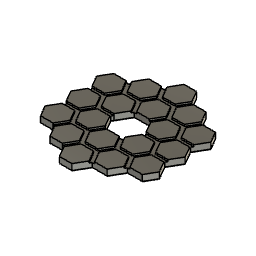
Mirror-v03 v3 (Autodesk Fusion 360 design; units mm, degrees)
Autodesk Fusion 360 part; units mm, degrees
sketch "Skizze1" plane through (0, 0, 0) normal (0, 0, 1) x (1, 0, 0)
  line L0 (8.3699, -6.8911) -> (9.0627, -6.8911)
  line L1 (23.8717, -11.2411) -> (21.7067, -7.4911) construction
  line L2 (4.3862, -7.4911) -> (2.2211, -11.2411) construction
  line L3 (21.0139, -7.4911) -> (21.3603, -8.0911)
  line L4 (21.3603, -6.8911) -> (23.1789, -3.7411)
  line L5 (17.723, -6.8911) -> (21.3603, -6.8911) construction
  line L6 (10.8814, -3.7411) -> (8.7163, -7.4911) construction
  line L7 (11.2278, -3.1411) -> (14.8651, -3.1411) construction
  line L8 (15.2115, -3.7411) -> (10.8814, -3.7411) construction
  line L9 (16.6837, -7.4911) -> (14.8651, -4.3411) construction
  line L10 (21.3603, -8.0911) -> (17.723, -8.0911) construction
  line L11 (17.3765, -7.4911) -> (21.7067, -7.4911) construction
  line L12 (21.7067, -7.4911) -> (23.8717, -3.7411) construction
  line L13 (10.8814, -3.7411) -> (15.2115, -3.7411) construction
  line L14 (-3.5813, -7.4911) -> (-1.7626, -10.6411) construction
  line L15 (9.4091, -7.4911) -> (9.0627, -6.8911)
  line L16 (17.3765, -7.4911) -> (15.2115, -3.7411) construction
  line L17 (21.3603, -6.8911) -> (21.0139, -7.4911)
  line L18 (8.7163, -7.4911) -> (10.8814, -11.2411) construction
  line L19 (14.8651, -4.3411) -> (11.2278, -4.3411) construction
  line L20 (21.7067, -7.4911) -> (17.3765, -7.4911) construction
  line L21 (9.4091, -7.4911) -> (11.2278, -10.6411)
  line L22 (15.2115, -3.7411) -> (17.3765, -7.4911) construction
  line L23 (8.7163, -7.4911) -> (10.8814, -3.7411) construction
  line L24 (1.8747, -10.6411) -> (3.6933, -7.4911)
  line L25 (15.9043, -3.7411) -> (17.723, -6.8911) construction
  line L26 (-2.109, -11.2411) -> (-4.2741, -7.4911) construction
  line L27 (14.8651, -10.6411) -> (16.6837, -7.4911) construction
  line L28 (10.8814, 3.7589) -> (8.7163, 0.0089) construction
  line L29 (-8.2578, -8.0911) -> (-10.0765, -11.2411)
  line L30 (17.723, -8.0911) -> (15.9043, -11.2411) construction
  line L31 (2.2211, -11.2411) -> (4.3862, -7.4911) construction
  line L32 (17.3765, -7.4911) -> (15.2115, -11.2411) construction
  line L33 (8.7163, 7.5089) -> (4.3862, 7.5089) construction
  line L34 (-8.6042, -7.4911) -> (-10.7693, -11.2411) construction
  line L35 (10.1885, 3.7589) -> (8.3699, 6.9089)
  line L36 (10.8814, -11.2411) -> (8.7163, -7.4911) construction
  line L37 (8.7163, -7.4911) -> (4.3862, -7.4911) construction
  line L38 (8.3699, -15.5911) -> (4.7326, -15.5911)
  line L39 (17.723, -0.5911) -> (15.9043, -3.7411) construction
  line L40 (8.7163, -22.4911) -> (4.3862, -22.4911) construction
  line L41 (4.3862, 0.0089) -> (8.7163, 0.0089) construction
  line L42 (4.7326, -21.8911) -> (8.3699, -21.8911) construction
  line L43 (4.7326, -6.8911) -> (8.3699, -6.8911)
  line L44 (9.4091, 0.0089) -> (11.2278, -3.1411) construction
  line L45 (10.8814, -3.7411) -> (8.7163, 0.0089) construction
  line L46 (4.3862, -22.4911) -> (8.7163, -22.4911) construction
  line L47 (8.3699, -23.0911) -> (4.7326, -23.0911) construction
  line L48 (23.1789, -3.7411) -> (21.3603, -0.5911)
  line L49 (10.1885, -3.7411) -> (8.3699, -0.5911) construction
  line L50 (11.2278, -10.6411) -> (11.5742, -11.2411)
  line L51 (-2.109, -18.7411) -> (-4.2741, -14.9911) construction
  line L52 (-2.8018, -18.7411) -> (-4.6205, -15.5911) construction
  line L53 (21.0139, -14.9911) -> (21.3603, -15.5911)
  line L54 (3.6933, -7.4911) -> (1.8747, -4.3411) construction
  line L55 (23.1789, -18.7411) -> (21.3603, -15.5911)
  line L56 (-4.2741, -14.9911) -> (-8.6042, -14.9911) construction
  line L57 (21.3603, -15.5911) -> (17.723, -15.5911) construction
  line L58 (17.3765, -14.9911) -> (15.2115, -11.2411) construction
  line L59 (15.9043, -11.2411) -> (17.723, -14.3911) construction
  line L60 (4.3759, -14.9895) -> (2.2081, -11.2411) construction
  line L61 (4.7326, -6.8911) -> (4.0398, -6.8911)
  line L62 (1.8595, -11.8154) -> (-1.7778, -11.8154) construction
  line L63 (17.3765, -22.4911) -> (21.7067, -22.4911) construction
  line L64 (-8.2578, -15.5911) -> (-10.0765, -18.7411)
  line L65 (4.3677, -22.5014) -> (2.2026, -18.7514) construction
  line L66 (16.6837, -14.9911) -> (14.8651, -11.8411) construction
  line L67 (8.7163, -14.9911) -> (10.8814, -18.7411) construction
  line L68 (8.3699, -29.3911) -> (10.1885, -26.2411)
  line L69 (4.3862, -7.4911) -> (2.2211, -3.7411) construction
  line L70 (10.1885, -26.2411) -> (8.3699, -23.0911) construction
  line L71 (8.7163, -14.9911) -> (10.8814, -11.2411) construction
  line L72 (14.8651, -25.6411) -> (16.6837, -22.4911)
  line L73 (17.723, -14.3911) -> (21.3603, -14.3911) construction
  line L74 (10.8814, -18.7411) -> (8.7163, -14.9911) construction
  line L75 (2.9139, -3.7411) -> (4.7326, -6.8911) construction
  line L76 (14.8651, -18.1411) -> (16.6837, -14.9911) construction
  line L77 (15.2115, -26.2411) -> (17.3765, -22.4911) construction
  line L78 (17.723, -15.5911) -> (15.9043, -18.7411) construction
  line L79 (-8.2578, -15.5911) -> (-7.9114, -14.9911)
  line L80 (1.8154, -18.1524) -> (3.6663, -14.948) construction
  line L81 (17.723, -21.8911) -> (21.3603, -21.8911)
  line L82 (21.3603, -14.3911) -> (23.1789, -11.2411)
  line L83 (10.1885, -26.2411) -> (10.5349, -25.6411)
  line L84 (9.4091, -22.4911) -> (11.2278, -25.6411) construction
  line L85 (17.0301, -21.8911) -> (16.6837, -22.4911)
  line L86 (-8.6042, 0.0089) -> (-10.7693, -3.7411) construction
  line L87 (4.7326, -15.5911) -> (4.0398, -15.5911)
  line L88 (8.7163, -29.9911) -> (10.8814, -26.2411) construction
  line L89 (11.2278, -25.6411) -> (10.5349, -25.6411)
  line L90 (-4.2741, 0.0089) -> (-2.109, -3.7411) construction
  line L91 (17.3765, -22.4911) -> (15.2115, -18.7411) construction
  line L92 (11.2278, -11.8411) -> (11.5742, -11.2411)
  line L93 (8.7163, -22.4911) -> (10.8814, -26.2411) construction
  line L94 (8.3699, -15.5911) -> (9.0627, -15.5911)
  line L95 (1.8747, -10.6411) -> (1.5282, -11.2411)
  line L96 (17.3765, -14.9911) -> (15.2115, -18.7411) construction
  line L97 (3.6933, -7.4911) -> (4.0398, -6.8911)
  line L98 (4.3862, 0.0089) -> (2.2211, -3.7411) construction
  line L99 (3.6663, -14.948) -> (1.8595, -11.8154)
  line L100 (2.2127, -18.7479) -> (4.3759, -14.9895) construction
  line L101 (10.8814, -26.2411) -> (8.7163, -22.4911) construction
  line L102 (2.2211, -3.7411) -> (4.3862, -7.4911) construction
  line L103 (15.2115, -18.7411) -> (17.3765, -22.4911) construction
  line L104 (15.2115, -11.2411) -> (17.3765, -14.9911) construction
  line L105 (-8.2578, -0.5911) -> (-10.0765, -3.7411)
  line L106 (17.3765, -14.9911) -> (21.7067, -14.9911) construction
  line L107 (-2.109, -11.2411) -> (2.2211, -11.2411) construction
  line L108 (2.2081, -11.2411) -> (-2.096, -11.2411) construction
  line L109 (11.2278, -18.1411) -> (14.8651, -18.1411) construction
  line L110 (-8.6042, -14.9911) -> (-10.7693, -18.7411) construction
  line L111 (11.2278, -19.3411) -> (9.4091, -22.4911) construction
  line L112 (2.2211, -11.2411) -> (4.3862, -14.9911) construction
  line L113 (9.4091, -14.9911) -> (11.2278, -18.1411) construction
  line L114 (14.8651, -3.1411) -> (16.6837, 0.0089) construction
  line L115 (4.7326, 0.6089) -> (8.3699, 0.6089) construction
  line L116 (-3.6204, -15.0117) -> (-1.8049, -18.1518) construction
  line L117 (14.8651, -19.3411) -> (11.2278, -19.3411) construction
  line L118 (23.8717, -3.7411) -> (21.7067, 0.0089) construction
  line L119 (8.3699, -0.5911) -> (4.7326, -0.5911) construction
  line L120 (4.7326, -29.3911) -> (8.3699, -29.3911)
  line L121 (4.7326, -15.5911) -> (2.9139, -18.7411) construction
  line L122 (10.8814, -11.2411) -> (8.7163, -14.9911) construction
  line L123 (10.1885, -18.7411) -> (8.3699, -15.5911) construction
  line L124 (4.3862, -29.9911) -> (8.7163, -29.9911) construction
  line L125 (8.3699, 6.9089) -> (4.7326, 6.9089)
  line L126 (8.7163, 0.0089) -> (10.8814, -3.7411) construction
  line L127 (14.8651, -11.8411) -> (11.2278, -11.8411) construction
  line L128 (10.8814, -18.7411) -> (8.7163, -22.4911) construction
  line L129 (11.2278, -11.8411) -> (9.4091, -14.9911)
  line L130 (-2.8018, -3.7411) -> (-4.6205, -0.5911) construction
  line L131 (1.8747, -3.1411) -> (3.6933, 0.0089) construction
  line L132 (23.8717, -18.7411) -> (21.7067, -14.9911) construction
  line L133 (15.2115, -18.7411) -> (10.8814, -18.7411) construction
  line L134 (10.8814, -18.7411) -> (15.2115, -18.7411) construction
  line L135 (-4.2836, -15.045) -> (-2.1376, -18.7549) construction
  line L136 (11.2278, -10.6411) -> (14.8651, -10.6411) construction
  line L137 (15.2115, -3.7411) -> (17.3765, 0.0089) construction
  line L138 (11.2278, -25.6411) -> (14.8651, -25.6411)
  line L139 (8.3699, -21.8911) -> (10.1885, -18.7411) construction
  line L140 (1.8595, -11.8154) -> (1.5282, -11.2411)
  line L141 (8.7163, -22.4911) -> (10.8814, -18.7411) construction
  line L142 (9.0627, -15.5911) -> (9.4091, -14.9911)
  line L143 (3.6663, -14.948) -> (4.0398, -15.5911)
  line L144 (8.7163, -14.9911) -> (4.3862, -14.9911) construction
  line L145 (4.3862, -14.9911) -> (2.2211, -18.7411) construction
  line L146 (10.8814, -26.2411) -> (15.2115, -26.2411) construction
  line L147 (10.8814, -11.2411) -> (15.2115, -11.2411) construction
  line L148 (8.7163, 0.0089) -> (4.3862, 0.0089) construction
  line L149 (2.2211, -3.7411) -> (4.3862, 0.0089) construction
  line L150 (4.3862, -7.4911) -> (8.7163, -7.4911) construction
  line L151 (4.3862, -14.9911) -> (8.7163, -14.9911) construction
  line L152 (15.2115, -11.2411) -> (10.8814, -11.2411) construction
  line L153 (17.3765, 0.0089) -> (15.2115, -3.7411) construction
  line L154 (-2.109, -3.7411) -> (-4.2741, -7.4911) construction
  line L155 (-10.7693, -11.2411) -> (-8.6042, -14.9911) construction
  line L156 (4.7326, -0.5911) -> (2.9139, -3.7411) construction
  line L157 (-8.2578, -6.8911) -> (-7.9114, -7.4911)
  line L158 (4.3862, 0.0089) -> (2.2211, 3.7589) construction
  line L159 (-2.1275, -26.2514) -> (2.2026, -26.2514) construction
  line L160 (-1.8049, -18.1518) -> (1.8154, -18.1524) construction
  line L161 (21.3603, -21.8911) -> (23.1789, -18.7411)
  line L162 (4.3862, -22.4911) -> (2.2211, -26.2411) construction
  line L163 (-8.6042, -14.9911) -> (-4.2741, -14.9911) construction
  line L164 (-4.6205, -15.5911) -> (-8.2578, -15.5911) construction
  line L165 (-1.7778, -11.8154) -> (-3.6204, -15.0117) construction
  line L166 (-10.0765, -11.2411) -> (-8.2578, -14.3911)
  line L167 (15.2115, -18.7411) -> (17.3765, -14.9911) construction
  line L168 (-4.2741, -22.4911) -> (-2.109, -18.7411) construction
  line L169 (-2.096, -11.2411) -> (-4.2836, -15.045) construction
  line L170 (15.9043, -18.7411) -> (17.723, -21.8911) construction
  line L171 (-10.0765, -3.7411) -> (-8.2578, -6.8911)
  line L172 (21.7067, -14.9911) -> (17.3765, -14.9911) construction
  line L173 (1.8747, -4.3411) -> (-1.7626, -4.3411) construction
  line L174 (2.2211, -3.7411) -> (-2.109, -3.7411) construction
  line L175 (-4.2741, -7.4911) -> (-8.6042, -7.4911) construction
  line L176 (17.723, -21.8911) -> (17.0301, -21.8911)
  line L177 (2.2211, -26.2411) -> (4.3862, -29.9911) construction
  line L178 (-4.6205, -8.0911) -> (-8.2578, -8.0911) construction
  line L179 (-1.7726, -25.6367) -> (1.8478, -25.6367)
  line L180 (21.7067, -22.4911) -> (23.8717, -18.7411) construction
  line L181 (-7.9114, -14.9911) -> (-8.2578, -14.3911)
  line L182 (-1.7626, -10.6411) -> (1.8747, -10.6411) construction
  line L183 (-3.5813, 0.0089) -> (-1.7626, -3.1411) construction
  line L184 (-3.5828, -22.5014) -> (-1.7726, -25.6367)
  line L185 (-4.2741, -14.9911) -> (-2.109, -11.2411) construction
  line L186 (-2.1376, -18.7549) -> (2.2127, -18.7479) construction
  line L187 (21.7067, -14.9911) -> (23.8717, -11.2411) construction
  line L188 (2.9139, -26.2411) -> (4.7326, -29.3911)
  line L189 (-2.109, -3.7411) -> (2.2211, -3.7411) construction
  line L190 (3.6579, -22.5014) -> (1.8478, -19.366) construction
  line L191 (1.8478, -25.6367) -> (3.6579, -22.5014) construction
  line L192 (-8.2578, -21.8911) -> (-4.6205, -21.8911)
  line L193 (-4.6205, -21.8911) -> (-2.8018, -18.7411) construction
  line L194 (2.2211, -18.7411) -> (4.3862, -22.4911) construction
  line L195 (16.6837, -22.4911) -> (14.8651, -19.3411) construction
  line L196 (-1.7626, -4.3411) -> (-3.5813, -7.4911) construction
  line L197 (1.8478, -19.366) -> (-1.7726, -19.366) construction
  line L198 (2.2211, 3.7589) -> (-2.109, 3.7589) construction
  line L199 (4.7326, -23.0911) -> (2.9139, -26.2411) construction
  line L200 (-2.109, -3.7411) -> (-4.2741, 0.0089) construction
  line L201 (21.3603, -14.3911) -> (21.0139, -14.9911)
  line L202 (-4.6205, -14.3911) -> (-2.8018, -11.2411) construction
  line L203 (2.2026, -26.2514) -> (4.3677, -22.5014) construction
  line L204 (-8.2578, -14.3911) -> (-4.6205, -14.3911) construction
  line L205 (-8.2578, -6.8911) -> (-4.6205, -6.8911) construction
  line L206 (2.9139, -18.7411) -> (4.7326, -21.8911) construction
  line L207 (2.9139, 3.7589) -> (4.7326, 0.6089) construction
  line L208 (-10.0765, -18.7411) -> (-8.2578, -21.8911)
  line L209 (-10.7693, -18.7411) -> (-8.6042, -22.4911) construction
  line L210 (4.7326, 6.9089) -> (2.9139, 3.7589)
  line L211 (-4.2741, -7.4911) -> (-2.109, -3.7411) construction
  line L212 (-8.6042, -7.4911) -> (-4.2741, -7.4911) construction
  line L213 (-2.1275, -18.7514) -> (-4.2926, -22.5014) construction
  line L214 (-4.2741, 0.0089) -> (-8.6042, 0.0089) construction
  line L215 (2.2211, 3.7589) -> (4.3862, 0.0089) construction
  line L216 (-1.7626, -3.1411) -> (1.8747, -3.1411) construction
  line L217 (-4.6205, -0.5911) -> (-3.9277, -0.5911)
  line L218 (-10.7693, -3.7411) -> (-8.6042, -7.4911) construction
  line L219 (-4.6205, -0.5911) -> (-8.2578, -0.5911)
  line L220 (-3.9377, -21.8867) -> (-3.5828, -22.5014)
  line L221 (1.8747, 3.1589) -> (-1.7626, 3.1589)
  line L222 (-7.9114, -7.4911) -> (-8.2578, -8.0911)
  line L223 (4.3862, 7.5089) -> (2.2211, 3.7589) construction
  line L224 (-3.5813, 0.0089) -> (-3.9277, -0.5911)
  line L225 (-3.9377, -21.8867) -> (-4.6205, -21.8911)
  line L226 (-2.109, 3.7589) -> (-4.2741, 0.0089) construction
  line L227 (-1.7726, -19.366) -> (-3.5828, -22.5014) construction
  line L228 (2.9139, -26.2411) -> (2.5613, -25.6302)
  line L229 (2.9139, 3.7589) -> (2.5675, 3.1589)
  line L230 (-1.7626, 3.1589) -> (-3.5813, 0.0089)
  line L231 (2.2026, -18.7514) -> (-2.1275, -18.7514) construction
  line L232 (3.6933, 0.0089) -> (1.8747, 3.1589) construction
  line L233 (-8.6042, -22.4911) -> (-4.2741, -22.4911) construction
  line L234 (-4.2926, -22.5014) -> (-2.1275, -26.2514) construction
  line L235 (1.8747, 3.1589) -> (2.5675, 3.1589)
  line L236 (1.8478, -25.6367) -> (2.5613, -25.6302)
  line L237 (-4.6205, -6.8911) -> (-2.8018, -3.7411)
  line L238 (23.1789, -11.2411) -> (21.3603, -8.0911)
  line L239 (11.2278, 3.1589) -> (10.5349, 3.1589)
  line L240 (16.6837, 0.0089) -> (17.0301, -0.5911)
  line L241 (16.6837, 0.0089) -> (14.8651, 3.1589)
  line L242 (11.2278, 3.1589) -> (9.4091, 0.0089) construction
  line L243 (10.8814, 3.7589) -> (8.7163, 7.5089) construction
  line L244 (-2.8018, -11.2411) -> (-4.6205, -8.0911) construction
  line L245 (15.2115, -11.2411) -> (17.3765, -7.4911) construction
  line L246 (21.7067, 0.0089) -> (17.3765, 0.0089) construction
  line L247 (14.8651, 3.1589) -> (11.2278, 3.1589)
  line L248 (-4.2741, -7.4911) -> (-2.109, -11.2411) construction
  line L249 (10.1885, 3.7589) -> (10.5349, 3.1589)
  line L250 (17.3765, 0.0089) -> (15.2115, 3.7589) construction
  line L251 (17.0301, -0.5911) -> (17.723, -0.5911)
  line L252 (8.3699, 0.6089) -> (10.1885, 3.7589) construction
  line L253 (15.2115, 3.7589) -> (10.8814, 3.7589) construction
  line L254 (21.3603, -0.5911) -> (17.723, -0.5911)
  line L255 (11.2278, -4.3411) -> (9.4091, -7.4911) construction
  line L256 (8.3699, -6.8911) -> (10.1885, -3.7411) construction
  line L257 (8.7163, 0.0089) -> (10.8814, 3.7589) construction
  line L258 (8.3699, 6.9089) -> (4.7326, 6.9089)
  line L259 (4.7326, 6.9089) -> (2.9139, 3.7589)
  line L260 (2.9139, 3.7589) -> (4.7326, 0.6089)
  line L261 (4.7326, 0.6089) -> (8.3699, 0.6089)
  line L262 (8.3699, 0.6089) -> (10.1885, 3.7589)
  line L263 (10.1885, 3.7589) -> (8.3699, 6.9089)
  line L264 (14.8651, 3.1589) -> (11.2278, 3.1589)
  line L265 (11.2278, 3.1589) -> (9.4091, 0.0089)
  line L266 (9.4091, 0.0089) -> (11.2278, -3.1411)
  line L267 (11.2278, -3.1411) -> (14.8651, -3.1411)
  line L268 (14.8651, -3.1411) -> (16.6837, 0.0089)
  line L269 (16.6837, 0.0089) -> (14.8651, 3.1589)
  line L270 (21.3603, -0.5911) -> (17.723, -0.5911)
  line L271 (17.723, -0.5911) -> (15.9043, -3.7411)
  line L272 (15.9043, -3.7411) -> (17.723, -6.8911)
  line L273 (17.723, -6.8911) -> (21.3603, -6.8911)
  line L274 (21.3603, -6.8911) -> (23.1789, -3.7411)
  line L275 (23.1789, -3.7411) -> (21.3603, -0.5911)
  line L276 (23.1789, -11.2411) -> (21.3603, -8.0911)
  line L277 (21.3603, -8.0911) -> (17.723, -8.0911)
  line L278 (17.723, -8.0911) -> (15.9043, -11.2411)
  line L279 (15.9043, -11.2411) -> (17.723, -14.3911)
  line L280 (17.723, -14.3911) -> (21.3603, -14.3911)
  line L281 (21.3603, -14.3911) -> (23.1789, -11.2411)
  line L282 (23.1789, -18.7411) -> (21.3603, -15.5911)
  line L283 (21.3603, -15.5911) -> (17.723, -15.5911)
  line L284 (17.723, -15.5911) -> (15.9043, -18.7411)
  line L285 (15.9043, -18.7411) -> (17.723, -21.8911)
  line L286 (17.723, -21.8911) -> (21.3603, -21.8911)
  line L287 (21.3603, -21.8911) -> (23.1789, -18.7411)
  line L288 (16.6837, -22.4911) -> (14.8651, -19.3411)
  line L289 (14.8651, -19.3411) -> (11.2278, -19.3411)
  line L290 (11.2278, -19.3411) -> (9.4091, -22.4911)
  line L291 (9.4091, -22.4911) -> (11.2278, -25.6411)
  line L292 (11.2278, -25.6411) -> (14.8651, -25.6411)
  line L293 (14.8651, -25.6411) -> (16.6837, -22.4911)
  line L294 (16.6837, -14.9911) -> (14.8651, -11.8411)
  line L295 (14.8651, -11.8411) -> (11.2278, -11.8411)
  line L296 (11.2278, -11.8411) -> (9.4091, -14.9911)
  line L297 (9.4091, -14.9911) -> (11.2278, -18.1411)
  line L298 (11.2278, -18.1411) -> (14.8651, -18.1411)
  line L299 (14.8651, -18.1411) -> (16.6837, -14.9911)
  line L300 (16.6837, -7.4911) -> (14.8651, -4.3411)
  line L301 (14.8651, -4.3411) -> (11.2278, -4.3411)
  line L302 (11.2278, -4.3411) -> (9.4091, -7.4911)
  line L303 (9.4091, -7.4911) -> (11.2278, -10.6411)
  line L304 (11.2278, -10.6411) -> (14.8651, -10.6411)
  line L305 (14.8651, -10.6411) -> (16.6837, -7.4911)
  line L306 (8.3699, -6.8911) -> (10.1885, -3.7411)
  line L307 (10.1885, -3.7411) -> (8.3699, -0.5911)
  line L308 (8.3699, -0.5911) -> (4.7326, -0.5911)
  line L309 (4.7326, -0.5911) -> (2.9139, -3.7411)
  line L310 (2.9139, -3.7411) -> (4.7326, -6.8911)
  line L311 (4.7326, -6.8911) -> (8.3699, -6.8911)
  line L312 (-1.7626, -3.1411) -> (1.8747, -3.1411)
  line L313 (1.8747, -3.1411) -> (3.6933, 0.0089)
  line L314 (3.6933, 0.0089) -> (1.8747, 3.1589)
  line L315 (1.8747, 3.1589) -> (-1.7626, 3.1589)
  line L316 (-1.7626, 3.1589) -> (-3.5813, 0.0089)
  line L317 (-3.5813, 0.0089) -> (-1.7626, -3.1411)
  line L318 (-8.2578, -6.8911) -> (-4.6205, -6.8911)
  line L319 (-4.6205, -6.8911) -> (-2.8018, -3.7411)
  line L320 (-2.8018, -3.7411) -> (-4.6205, -0.5911)
  line L321 (-4.6205, -0.5911) -> (-8.2578, -0.5911)
  line L322 (-8.2578, -0.5911) -> (-10.0765, -3.7411)
  line L323 (-10.0765, -3.7411) -> (-8.2578, -6.8911)
  line L324 (-1.7626, -10.6411) -> (1.8747, -10.6411)
  line L325 (1.8747, -10.6411) -> (3.6933, -7.4911)
  line L326 (3.6933, -7.4911) -> (1.8747, -4.3411)
  line L327 (1.8747, -4.3411) -> (-1.7626, -4.3411)
  line L328 (-1.7626, -4.3411) -> (-3.5813, -7.4911)
  line L329 (-3.5813, -7.4911) -> (-1.7626, -10.6411)
  line L330 (-8.2578, -14.3911) -> (-4.6205, -14.3911)
  line L331 (-4.6205, -14.3911) -> (-2.8018, -11.2411)
  line L332 (-2.8018, -11.2411) -> (-4.6205, -8.0911)
  line L333 (-4.6205, -8.0911) -> (-8.2578, -8.0911)
  line L334 (-8.2578, -8.0911) -> (-10.0765, -11.2411)
  line L335 (-10.0765, -11.2411) -> (-8.2578, -14.3911)
  line L336 (-8.2578, -21.8911) -> (-4.6205, -21.8911)
  line L337 (-4.6205, -21.8911) -> (-2.8018, -18.7411)
  line L338 (-2.8018, -18.7411) -> (-4.6205, -15.5911)
  line L339 (-4.6205, -15.5911) -> (-8.2578, -15.5911)
  line L340 (-8.2578, -15.5911) -> (-10.0765, -18.7411)
  line L341 (-10.0765, -18.7411) -> (-8.2578, -21.8911)
  line L342 (1.8562, -25.6514) -> (3.6749, -22.5014)
  line L343 (3.6749, -22.5014) -> (1.8562, -19.3514)
  line L344 (1.8562, -19.3514) -> (-1.7811, -19.3514)
  line L345 (-1.7811, -19.3514) -> (-3.5997, -22.5014)
  line L346 (-3.5997, -22.5014) -> (-1.7811, -25.6514)
  line L347 (-1.7811, -25.6514) -> (1.8562, -25.6514)
  line L348 (4.7326, -23.0911) -> (2.9139, -26.2411)
  line L349 (2.9139, -26.2411) -> (4.7326, -29.3911)
  line L350 (4.7326, -29.3911) -> (8.3699, -29.3911)
  line L351 (8.3699, -29.3911) -> (10.1885, -26.2411)
  line L352 (10.1885, -26.2411) -> (8.3699, -23.0911)
  line L353 (8.3699, -23.0911) -> (4.7326, -23.0911)
  line L354 (2.9139, -18.7411) -> (4.7326, -21.8911)
  line L355 (4.7326, -21.8911) -> (8.3699, -21.8911)
  line L356 (8.3699, -21.8911) -> (10.1885, -18.7411)
  line L357 (10.1885, -18.7411) -> (8.3699, -15.5911)
  line L358 (8.3699, -15.5911) -> (4.7326, -15.5911)
  line L359 (4.7326, -15.5911) -> (2.9139, -18.7411)
  line L360 (1.8747, -18.1411) -> (3.6933, -14.9911)
  line L361 (3.6933, -14.9911) -> (1.8747, -11.8411)
  line L362 (1.8747, -11.8411) -> (-1.7626, -11.8411)
  line L363 (-1.7626, -11.8411) -> (-3.5813, -14.9911)
  line L364 (-3.5813, -14.9911) -> (-1.7626, -18.1411)
  line L365 (-1.7626, -18.1411) -> (1.8747, -18.1411)
  point P0 (13.0464, -7.4911)
  point P1 (6.5512, 3.7589)
  point P2 (19.5416, -3.7411)
  point P3 (19.5416, -11.2411)
  point P4 (13.0464, 0.0089)
  point P5 (6.5512, -3.7411)
  point P6 (0.0376, -22.5014)
  point P7 (6.5512, -26.2411)
  point P8 (6.5512, -18.7411)
  point P9 (19.5416, -3.7411)
  point P10 (13.0464, -7.4911)
  point P11 (6.5512, 6.9089)
  point P12 (19.5416, -11.2411)
  point P13 (6.5512, 3.7589)
  point P14 (13.0464, -22.4911)
  point P15 (0.056, 0.0089)
  point P16 (13.0464, -14.9911)
  point P17 (-6.4392, -18.7411)
  point P18 (0.056, 0.0089)
  point P19 (13.0464, 0.0089)
  point P20 (6.5512, -18.7411)
  point P21 (-6.4392, -11.2411)
  point P22 (6.5512, -11.2411)
  point P23 (19.5416, -18.7411)
  point P24 (13.0464, -14.9911)
  point P25 (6.5512, -11.2411)
  point P26 (0.056, -7.4911)
  point P27 (0.056, 0.0089)
  point P28 (-6.4392, -3.7411)
  point P29 (-6.4392, -11.2411)
  point P30 (-6.4392, -3.7411)
  point P31 (0.056, -7.4911)
  point P32 (6.5512, -3.7411)
  point P33 (19.5416, -18.7411)
  point P34 (-6.4392, -18.7411)
  point P35 (0.0376, -22.5014)
  point P36 (13.0464, -22.4911)
  point P37 (6.5512, -26.2411)
  point P38 (-6.4392, -11.2411)
  point P39 (6.5512, 3.7589)
  point P40 (13.0464, 0.0089)
  point P41 (19.5416, -3.7411)
  point P42 (19.5416, -11.2411)
  point P43 (19.5416, -18.7411)
  point P44 (13.0464, -22.4911)
  point P45 (13.0464, -14.9911)
  point P46 (13.0464, -7.4911)
  point P47 (6.5512, -3.7411)
  point P48 (0.056, 0.0089)
  point P49 (-6.4392, -3.7411)
  point P50 (0.056, -7.4911)
  point P51 (-6.4392, -11.2411)
  point P52 (-6.4392, -18.7411)
  point P53 (0.0376, -22.5014)
  point P54 (6.5512, -26.2411)
  point P55 (6.5512, -18.7411)
  point P56 (0.056, -14.9911)
  dimension "d1" = 7.5
  dimension "d10" = 6.3
  dimension "d12" = 6.3
  constraint horizontal L174
  constraint equal L8 L158
  constraint equal L28 L158
  constraint equal L8 L98
  constraint equal L8 L174
  constraint equal L8 L37
  constraint equal L34 L198
  constraint equal L198 L214
  constraint equal L60 L198
  constraint equal L101 L198
  constraint equal L51 L198
  constraint equal L65 L158
  constraint equal L20 L149
  constraint equal L144 L149
  constraint equal L128 L149
  constraint equal L149 L223
  constraint equal L122 L149
  constraint equal L149 L153
  constraint horizontal L56
  constraint horizontal L198
  constraint horizontal L8
  constraint horizontal L253
  constraint horizontal L148
  constraint horizontal L214
  constraint horizontal L40
  constraint horizontal L108
  constraint horizontal L37
  constraint horizontal L246
  constraint horizontal L152
  constraint horizontal L33
  constraint horizontal L133
  constraint horizontal L144
  constraint horizontal L20
  constraint horizontal L231
  constraint midpoint L90 L200
  constraint midpoint L174 L189
  constraint midpoint L98 L149
  constraint midpoint L6 L23
  constraint midpoint L37 L150
  constraint midpoint L8 L13
  constraint midpoint L137 L153
  constraint midpoint L147 L152
  constraint midpoint L107 L108
  constraint midpoint L144 L151
  constraint horizontal L175
  constraint midpoint L175 L212
  constraint midpoint L41 L148
  constraint coincident P48 P27
  constraint midpoint L56 L163
  constraint midpoint L186 L231
  constraint midpoint L40 L46
  constraint midpoint L133 L134
  constraint midpoint L11 L20
  constraint equal L172 L198
  constraint horizontal L172
  constraint midpoint L106 L172
  constraint coincident P39 P13
  constraint coincident P40 P19
  constraint coincident P41 P9
  constraint coincident P46 P10
  constraint coincident P42 P12
  constraint coincident P45 P24
  constraint coincident P25 P22
  constraint coincident P50 P31
  constraint coincident P49 P30
  constraint coincident P51 P38
  constraint coincident P20 P8
  constraint coincident P43 P33
  constraint coincident P47 P32
  constraint coincident P52 P34
  constraint coincident P53 P35
  constraint coincident P54 P37
  constraint coincident P44 P36
  constraint horizontal L125
  constraint horizontal L247
  constraint horizontal L254
  constraint horizontal L19
  constraint horizontal L10
  constraint horizontal L57
  constraint horizontal L127
  constraint horizontal L117
  constraint horizontal L47
  constraint horizontal L38
  constraint horizontal L119
  constraint horizontal L173
  constraint horizontal L197
  constraint horizontal L164
  constraint horizontal L219
  constraint horizontal L62
  constraint horizontal L178
  constraint horizontal L221
  constraint equal L125 L247
  constraint equal L221 L247
  constraint equal L115 L119
  constraint equal L114 L254
  constraint equal L7 L19
  constraint equal L5 L10
  constraint equal L127 L136
  constraint equal L54 L75
  constraint equal L130 L183
  constraint equal L178 L205
  constraint equal L62 L182
  constraint equal L164 L204
  constraint equal L160 L197
  constraint equal L42 L47
  constraint equal L109 L117
  constraint equal L57 L73
  constraint equal L38 L119
  constraint midpoint P11 L125
  constraint coincident L0.end L23
  constraint parallel L15 L21
  constraint coincident L61.end L69
  constraint parallel L43 L61
  constraint coincident L95.end L107
  constraint coincident L87.end L145
  constraint coincident L94.end L67
  constraint coincident L50.end L152
  constraint parallel L21 L50
  constraint parallel L129 L142
  constraint parallel L38 L87
  constraint parallel L99 L140
  constraint coincident L157.end L175
  constraint coincident L217.end L90
  constraint coincident L229.end L215
  constraint coincident L239.end L257
  constraint coincident L3.start L20
  constraint coincident L53.start L106
  constraint coincident L85.start L91
  constraint coincident L83.end L93
  constraint coincident L228.end L203
  constraint coincident L79.end L163
  constraint parallel L157 L171
  constraint parallel L217 L219
  constraint parallel L221 L235
  constraint parallel L35 L249
  constraint coincident L240.end L137
  constraint parallel L240 L241
  constraint parallel L4 L17
  constraint parallel L82 L201
  constraint parallel L81 L176
  constraint parallel L64 L79
  constraint coincident L220.start L213
  constraint parallel L184 L220
  constraint parallel L188 L228
  constraint parallel L89 L138
  constraint equal L263 L264
  constraint equal L264 L270
  constraint equal L270 L276
  constraint equal L276 L283
  constraint equal L334 L340
  constraint equal L340 L345
  constraint equal L345 L350
  constraint equal L287 L351
  constraint equal L311 L324
  constraint equal L295 L311
  constraint equal L295 L305
  constraint equal L277 L305
  constraint equal L290 L355
  constraint equal L290 L299
  constraint coincident P55 P20
  constraint equal L318 L333
  constraint equal L309 L312
  constraint equal L359 L362
  constraint collinear L67.start L112.end P56
  constraint collinear P50 P48 P56
  constraint horizontal L258
  constraint horizontal L315
  constraint horizontal L264
  constraint horizontal L308
  constraint horizontal L270
  constraint horizontal L301
  constraint horizontal L327
  constraint horizontal L321
  constraint horizontal L333
  constraint horizontal L277
  constraint horizontal L295
  constraint horizontal L358
  constraint horizontal L362
  constraint horizontal L339
  constraint horizontal L344
  constraint horizontal L353
  constraint horizontal L289
  constraint horizontal L283
  measures "d1" distance of L90 L158
  measures "d10" distance of L35 L207
  measures "d12" distance of L259 L262
extrude "Extrusion1" add sketch "Skizze1" against normal blind 2 contours L43 L306 L307 L308 L309 L310 L311 | L21 L300 L301 L302 L303 L304 L305 | L24 L324 L325 L326 L327 L328 L329 | L129 L294 L295 L296 L297 L298 L299 | L99 L143 L360 L361 L362 L363 L364 L365 | L38 L354 L355 L356 L357 L358 L359 | L3 L17 L53 L79 L83 L85 L89 L157 L176 L181 L201 L217 L220 L222 L224 L225 L228 L229 L235 L236 L237 L239 L240 L249 L251 L260 L261 L262 L265 L266 L267 L268 L271 L272 L273 L277 L278 L279 L280 L283 L284 L285 L288 L289 L290 L291 L312 L313 L314 L317 L318 L319 L320 L330 L331 L332 L333 L337 L338 L339 L342 L343 L344 L345 L348 L352 L353 | L82 L238 L276 L277 L278 L279 L280 L281 | L4 L48 L254 L270 L271 L272 L273 L274 L275 | L55 L81 L161 L282 L283 L284 L285 L286 L287 | L241 L247 L264 L265 L266 L267 L268 L269 | L72 L138 L288 L289 L290 L291 L292 L293 | L35 L125 L210 L258 L259 L260 L261 L262 L263 | L68 L120 L188 L348 L349 L350 L351 L352 L353 | L221 L230 L312 L313 L314 L315 L316 L317 | L179 L184 L220 L236 L342 L343 L344 L345 | L105 L171 L219 L237 L318 L319 L320 L321 L322 L323 | L29 L166 L330 L331 L332 L333 L334 L335 | L64 L192 L208 L336 L337 L338 L339 L340 L341
fillet "Abrundung1" radius 0.25 1 faces at (7.1554, -22.2874, -2)
extrude "Extrusion2" cut sketch "Skizze1" against normal blind 0.5 contours L3 L17 L53 L79 L83 L85 L89 L157 L176 L181 L201 L217 L220 L222 L224 L225 L228 L229 L235 L236 L237 L239 L240 L249 L251 L260 L261 L262 L265 L266 L267 L268 L271 L272 L273 L277 L278 L279 L280 L283 L284 L285 L288 L289 L290 L291 L312 L313 L314 L317 L318 L319 L320 L330 L331 L332 L333 L337 L338 L339 L342 L343 L344 L345 L348 L352 L353
equation "d10 = d1 - 1.2 mm"
equation "d12 = d10"
